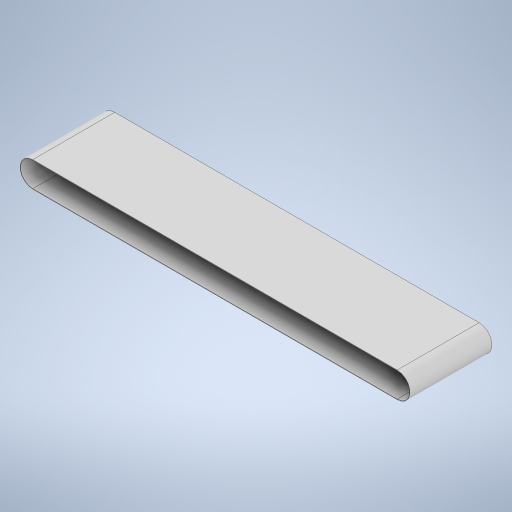
# Autodesk Inventor part: BandaLona
Saved by Autodesk Inventor 2024 (Build 280153000, 153)
## iProperties
Created: 2024-06-28
Part Number: BandaLona
Material: Genérico
Document SubType Name: Modeling
Designer: USER
Density: 1 g/cm^3
Appearance: Valor por defecto
Author: USER
Autodesk Inventor part; units mm, degrees
ref_plane "YZ Plane" through (0, 0, 0) normal (1, 0, 0) x (0, 1, 0)
ref_plane "XZ Plane" through (0, 0, 0) normal (0, 1, 0) x (-1, 0, 0)
ref_plane "XY Plane" through (0, 0, 0) normal (0, 0, 1) x (1, 0, 0)
sketch "Boceto1" plane through (0, 0, 0) normal (0, 0, 1) x (1, 0, 0)
  line L0 (-1900, -437.5529) -> (2550, -437.5529)
  line L1 (2550, -137.5529) -> (-1900, -137.5529)
  line L2 (-2050, -137.5529) -> (-1900, -137.5529) construction
  line L3 (-4000, 3228.1666) -> (2700, 3528.1666) construction
  line L4 (750, 6893.8862) -> (-2050, -137.5529) construction
  arc A0 (2550, -437.5529) -> (2550, -137.5529) centre (2550, -287.5529) ccw
  arc A1 (-1900, -137.5529) -> (-1900, -437.5529) centre (-1900, -287.5529) ccw
  arc A2 (-1900, -130.5529) -> (-1900, -444.5529) centre (-1900, -287.5529) ccw
  line L5 (-1900, -444.5529) -> (2550, -444.5529)
  arc A3 (2550, -444.5529) -> (2550, -130.5529) centre (2550, -287.5529) ccw
  line L6 (2550, -130.5529) -> (-1900, -130.5529)
  point P0 (-650, 3378.1666)
  point P1 (2700, -287.5529)
  point P2 (-2050, -287.5529)
  dimension "d5" = 6000
  dimension "d6" = 300
  dimension "d7" = 7
  dimension "d9" = 0
  dimension "d10" = 0
  constraints: 14 end point, 11 point on circle, 5 tangent, 4 centre point, 2 midpoint, 2 parallel, 1 horizontal, 3 other
  measures "d5" distance of L2.start L3.end
  measures "d6" distance between parallel lines of L0 L1
  measures "d7" distance between parallel lines of L1 L6
  measures "d9" horizontal distance of L3.end point (2700, -287.553)
  measures "d10" horizontal distance of L2.start point (-2050, -287.553)
extrude "Extrusión1" add sketch "Boceto1" along normal blind 1000
equation "\"d5\" = L"
equation "\"L\" = 6000"
